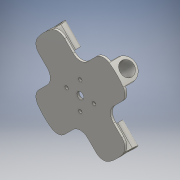
# Autodesk Inventor part: Boom Platform
Saved by Autodesk Inventor 2016 (Build 200138000, 138)
## iProperties
Created: 2016-01-01
Part Number: Boom Platform
Material: Generic
Document SubType Name: Modeling
Designer: jonathan
Density: 1 g/cm^3
Appearance: Steel
Author: jonathan
Autodesk Inventor part; units mm, degrees
ref_plane "YZ Plane" through (0, 0, 0) normal (1, 0, 0) x (0, 1, 0)
ref_plane "XZ Plane" through (0, 0, 0) normal (0, 1, 0) x (-1, 0, 0)
ref_plane "XY Plane" through (0, 0, 0) normal (0, 0, 1) x (1, 0, 0)
sketch "Sketch1" plane through (0, 0, 0) normal (0, 1, 0) x (-1, 0, 0)
  circle A0 centre (0, 0) radius 75
  circle A1 centre (0, 0) radius 5
  dimension "d0" = 150
  dimension "d3" = 10
  constraints: 2 centre point, 2 coincident
  measures "d0" diameter of A0
  measures "d3" diameter of A1
extrude "Extrusion2" add sketch "Sketch1" along normal blind 3
sketch "Sketch3" plane through (0, 3, 0) normal (0, 1, 0) x (1, 0, 0)
  circle A0 centre (0, 0) radius 75 projected
  line L0 (0, 0) -> (-53.033, 53.033)
  line L1 (0, 0) -> (0, 53.033)
  line L2 (-30.7483, 30.7483) -> (-20.1417, 41.3549)
  line L3 (-20.1417, 41.3549) -> (-41.3549, 62.5681)
  line L4 (-30.7483, 30.7483) -> (-41.3549, 20.1417)
  line L5 (-41.3549, 20.1417) -> (-62.5681, 41.3549)
  arc A1 (-42.1189, 62.0564) -> (-62.5681, 41.3549) centre (0, 0) ccw
  dimension "d12" = 45
  dimension "d22" = 30
  dimension "d23" = 15
  constraints: 12 end point, 5 point on circle, 2 equal length, 2 perpendicular, 2 point on line, 1 centre point, 1 coincident, 1 vertical
  measures "d12" angle of L1 L0
  measures "d22" distance of L2.end L3.end
  measures "d23" distance of L2.start L2.end
extrude "Extrusion3" add sketch "Sketch3" along normal blind 25 contours L3 L2 L0 A0 | A0 L0 L4 L5
fillet "Fillet1" radius 15 2 edges at (-30.7483, 28, -51.9615) (-51.9615, 28, -30.7483)
sketch "Sketch5" plane through (-41.3549, 3, -20.1417) normal (0.7071068, 0, 0.7071068) x (0.7071068, 0, -0.7071068)
  circle A0 centre (15, 12) radius 10
  line L0 (15, -3) -> (15, 12)
  dimension "d16" = 20
  dimension "d24" = 15
  constraints: 2 end point, 1 centre point, 1 vertical
  measures "d16" diameter of A0
  measures "d24" distance of L0.start L0.end
extrude "Extrusion4" cut sketch "Sketch5" against normal through all
pattern_circular "Circular Pattern1" count 4 over 360 about axis through (0, 0, 0) along (0, 1, 0) of "Extrusion3", "Extrusion4", "Fillet1"
sketch "Sketch6" plane through (0, 3, 0) normal (0, 1, 0) x (1, 0, 0)
  circle A0 centre (0, -20) radius 2.5
  circle A1 centre (20, 0) radius 2.5
  circle A2 centre (0, 20) radius 2.5
  circle A3 centre (-20, 0) radius 2.5
  point P0 (0, 0)
  dimension "d25" = 20
  dimension "d26" = 5
  dimension "d29" = 360
  constraints: 4 centre point, 9 other
  measures "d25" distance of A0.centre point (0, 0)
  measures "d26" diameter of A0
extrude "Extrusion5" cut sketch "Sketch6" against normal through all
sketch "Sketch7" plane through (0, 3, 0) normal (0, 1, 0) x (1, 0, 0)
  line L0 (0, 0) -> (75, 0)
  circle A0 centre (0, 0) radius 75 projected
  line L1 (37.5, 0) -> (68.3578, -30.8578)
  line L2 (37.5, 0) -> (68.3578, 30.8578)
  arc A1 (68.3578, -30.8578) -> (68.3578, 30.8578) centre (0, 0) ccw
  line L3 (0, 37.5) -> (-30.8578, 68.3578)
  line L4 (0, 0) -> (0, 75)
  line L5 (0, 37.5) -> (30.8578, 68.3578)
  arc A2 (30.8578, 68.3578) -> (-30.8578, 68.3578) centre (0, 0) ccw
  line L6 (-37.5, 0) -> (-68.3578, -30.8578)
  line L7 (0, 0) -> (-75, 0)
  line L8 (-37.5, 0) -> (-68.3578, 30.8578)
  arc A3 (-68.3578, 30.8578) -> (-68.3578, -30.8578) centre (0, 0) ccw
  line L9 (0, -37.5) -> (30.8578, -68.3578)
  line L10 (0, 0) -> (0, -75)
  line L11 (0, -37.5) -> (-30.8578, -68.3578)
  arc A4 (-30.8578, -68.3578) -> (30.8578, -68.3578) centre (0, 0) ccw
  dimension "d33" = 45
  dimension "d34" = 45
  dimension "d37" = 360
  constraints: 24 end point, 11 point on circle, 4 centre point, 1 coincident, 1 horizontal, 1 midpoint, 41 other
  measures "d33" angle of L1 L0
  measures "d34" angle of L2 L0
extrude "Extrusion6" cut sketch "Sketch7" against normal blind 25 contours L2 A0 L0 | L0 A0 L1 | L3 A0 L4 | L4 A0 L5 | L6 A0 L7 | L7 A0 L8 | L9 A0 L10 | L10 A0 L11
fillet "Fillet2" radius 15 4 edges at (0, 1.5, -37.5) (37.5, 1.5, 0) (0, 1.5, 37.5) (-37.5, 1.5, 0)
fillet "Fillet3" radius 15 8 edges at (-30.8578, 1.5, 68.3578) (-68.3578, 1.5, 30.8578) (30.8578, 1.5, 68.3578) (68.3578, 1.5, 30.8578) (68.3578, 1.5, -30.8578) (30.8578, 1.5, -68.3578) (-30.8578, 1.5, -68.3578) (-68.3578, 1.5, -30.8578)
body "Solid2"
